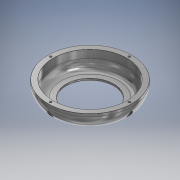
# Autodesk Inventor part: top cover 2
Saved by Autodesk Inventor 2022 (Build 260153000, 153)
## iProperties
Created: 2018-05-09
Part Number: top cover 2
Material: Aluminum 6061
Document SubType Name: Modeling
Designer: SimonD
Density: 2.7 g/cm^3
Appearance: Machined - Aluminum
Author: SimonD
Autodesk Inventor part; units mm, degrees
ref_plane "YZ Plane" through (0, 0, 0) normal (1, 0, 0) x (0, 1, 0)
ref_plane "XZ Plane" through (0, 0, 0) normal (0, 1, 0) x (-1, 0, 0)
ref_plane "XY Plane" through (0, 0, 0) normal (0, 0, 1) x (1, 0, 0)
sketch "Sketch1" plane through (0, 0, 0) normal (0, 0, 1) x (1, 0, 0)
  circle A0 centre (0, 0) radius 80
  dimension "d0" = 160
  constraints: 1 centre point, 1 coincident
  measures "d0" diameter of A0
extrude "Extrusion1" add sketch "Sketch1" along normal blind 35
sketch "Sketch2" plane through (0, 0, 35) normal (0, 0, 1) x (1, 0, 0)
  circle A0 centre (0, 0) radius 45
  dimension "d3" = 90
  constraints: 1 centre point, 1 coincident
  measures "d3" diameter of A0
extrude "Extrusion2" cut sketch "Sketch2" against normal blind 35
sketch "Sketch3" plane through (0, 0, 35) normal (0, 0, 1) x (1, 0, 0)
  circle A0 centre (0, 0) radius 70
  dimension "d6" = 140
  constraints: 1 centre point, 1 coincident
  measures "d6" diameter of A0
extrude "Extrusion3" cut sketch "Sketch3" against normal blind 30
fillet "Fillet4" radius 15 1 edges at (-70, 0, 5)
fillet "Fillet6" radius 30 1 edges at (-80, 0, 0)
sketch "Sketch6" plane through (0, 0, 35) normal (0, 0, 1) x (1, 0, 0)
  point P0 (0, 0)
  point P1 (0, 75)
  point P2 (-75, 0)
  point P3 (0, -75)
  point P4 (75, 0)
  dimension "d35" = 75
  dimension "d36" = 75
  dimension "d37" = 75
  dimension "d38" = 0
  dimension "d39" = 75
  measures "d35" distance of point (0, 75) point (0, 0)
  measures "d36" distance of point (-75, 0) point (0, 0)
  measures "d37" distance of point (0, -75) point (0, 0)
  measures "d38" horizontal distance of point (0, -75) point (0, 0)
  measures "d39" distance of point (75, 0) point (0, 0)
hole "Hole2" at (0, 75, 35) at (-75, 0, 35) at (0, -75, 35) at (75, 0, 35) direction (0, 0, -1) diameter 4 end through all
sketch "Sketch7" plane through (0, 0, 0) normal (0, 0, -1) x (-1, 0, 0)
  circle A0 centre (0, -75) radius 2 projected
  circle A1 centre (0, -75) radius 4
  circle A2 centre (75, 0) radius 2 projected
  circle A3 centre (75, 0) radius 4
  circle A4 centre (0, 75) radius 2 projected
  circle A5 centre (0, 75) radius 4
  circle A6 centre (-75, 0) radius 2 projected
  circle A7 centre (-75, 0) radius 4
  point P0 (0, 0)
  dimension "d50" = 8
  dimension "d51" = 8
  dimension "d52" = 8
  dimension "d53" = 8
  constraints: 4 centre point, 4 coincident
  measures "d50" diameter of A1
  measures "d51" diameter of A3
  measures "d52" diameter of A5
  measures "d53" diameter of A7
extrude "Extrusion5" cut sketch "Sketch7" against normal blind 22.5 contours A0 | A1 | A2 | A3 | A4 | A5 | A6 | A7
fillet "Fillet8" radius 2 1 edges at (-45, 0, 0)
chamfer "Chamfer3" distance 0.1 angle 45 8 edges at (-3.0942, 77.5349, 18.2345) (3.7774, 73.6843, 11.7118) (75.8369, 3.9115, 14.9256) (75.8118, -3.9168, 14.8831) (-71.0002, -0.0437, 8.576) (-78.9995, -0.0448, 22.3171) (3.785, -73.7064, 11.7409) (-3.1203, -77.5027, 18.1618)
chamfer "Chamfer4" distance 0.25 angle 45 3 edges at (-80, 0, 35) (-70, 0, 35) (-45, 0, 5)
sketch "Sketch8" plane through (0, 0, 0) normal (0, 0, -1) x (-1, 0, 0)
  point P0 (0, 0)
  point P1 (-48, 0)
  point P2 (0, -48)
  point P3 (48, 0)
  point P4 (0, 48)
  dimension "d66" = 48
  dimension "d67" = 48
  dimension "d68" = 48
  dimension "d69" = 48
  measures "d66" distance of point (-48, 0) point (0, 0)
  measures "d67" distance of point (0, 48) point (0, 0)
  measures "d68" distance of point (48, 0) point (0, 0)
  measures "d69" distance of point (0, 0) point (0, -48)
hole "Hole3" [suppressed]
body "Solid1"
